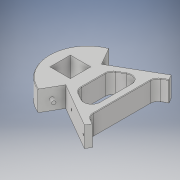
# Autodesk Inventor part: Profil_Winkel
Saved by Autodesk Inventor 2019 (Build 230136000, 136)
## iProperties
Created: 2018-08-17
Part Number: Profil_Winkel
Material: Generic
Document SubType Name: Modeling
Designer: Julia
Density: 1 g/cm^3
Appearance: Default
Author: Julia
Autodesk Inventor part; units mm, degrees
ref_plane "YZ Plane" through (0, 0, 0) normal (1, 0, 0) x (0, 1, 0)
ref_plane "XZ Plane" through (0, 0, 0) normal (0, 1, 0) x (-1, 0, 0)
ref_plane "XY Plane" through (0, 0, 0) normal (0, 0, 1) x (1, 0, 0)
sketch "Sketch1" plane through (0, 0, 0) normal (0, 1, 0) x (-1, 0, 0)
  line L0 (-126.3701, 48.161) -> (-51.2671, 4.8003) construction
  line L1 (-51.2671, 4.8003) -> (-126.3701, -38.5605) construction
  line L2 (-126.3701, -38.5605) -> (-126.3701, 48.161) construction
  line L3 (110.9585, 0) -> (-59.5814, 0) construction
  line L4 (83.2089, 69.641) -> (63.2089, 35)
  line L5 (63.2089, 35) -> (-23.3937, 85)
  line L6 (-23.3937, 85) -> (-29.3937, 74.6077)
  line L7 (-29.3937, 74.6077) -> (-12.0731, 64.6077)
  line L8 (0.9172, 57.1077) -> (44.2185, 32.1077)
  line L9 (83.2089, -69.641) -> (63.2089, -35)
  line L10 (63.2089, -35) -> (-23.3937, -85)
  line L11 (-23.3937, -85) -> (-29.3937, -74.6077)
  line L12 (-29.3937, -74.6077) -> (-12.0731, -64.6077)
  line L13 (0.9172, -57.1077) -> (44.2185, -32.1077)
  arc A0 (83.2089, -69.641) -> (83.2089, 69.641) centre (55.3678, 0) ccw
  line L14 (-12.0731, 64.6077) -> (-12.0731, -64.6077)
  line L15 (0.9172, 57.1077) -> (0.9172, -57.1077)
  line L16 (44.2185, 32.1077) -> (44.2185, -32.1077)
  dimension "d3" = 40
  dimension "d4" = 100
  dimension "d5" = 12
  dimension "d7" = 20
  dimension "d19" = 70
  dimension "d20" = 75
  dimension "d21" = 15
  dimension "d22" = 50
  constraints: 34 end point, 7 symmetric about line, 5 vertical, 4 perpendicular, 2 equal length, 2 horizontal, 2 point on circle, 1 centre point, 1 collinear, 1 parallel, 1 point on line, 3 other
  measures "d3" distance of L4.start L4.end
  measures "d4" distance of L4.end L5.end
  measures "d5" distance of L5.end L6.end
  measures "d7" distance of L6.end L7.end
  measures "d19" distance of L9.end L4.end
  measures "d20" radius of A0
  measures "d21" distance of L8.start L7.end
  measures "d22" distance of L8.start L8.end
extrude "Extrusion1" add sketch "Sketch1" along normal blind 40
sketch "Sketch2" plane through (-63.2089, 0, 35) normal (0.8660254, 0, 0.5) x (0.5, 0, -0.8660254)
  circle A0 centre (-20, 20) radius 3.4
  line L0 (-40, 40) -> (0, 40) projected
  line L1 (-40, 0) -> (-40, 40) projected
  point P0 (61.9153, 0)
  point P1 (-20, 40)
  point P2 (-40, 20)
  dimension "d10" = 6.8
  constraints: 2 midpoint, 1 centre point, 1 horizontal alignment, 1 vertical alignment
  measures "d10" diameter of A0
extrude "Extrusion2" add sketch "Sketch2" along normal blind 10
sketch "Sketch3" plane through (-83.2089, 0, -69.641) normal (0.8660254, 0, -0.5) x (-0.5, 0, -0.8660254)
  circle A0 centre (-20, 20) radius 3.4
  line L0 (-40, 40) -> (0, 40) projected
  line L1 (0, 0) -> (0, 40) projected
  point P0 (-101.9153, 0)
  point P1 (-20, 40)
  point P2 (0, 20)
  dimension "d13" = 6.8
  constraints: 2 midpoint, 1 centre point, 1 horizontal alignment, 1 vertical alignment
  measures "d13" diameter of A0
extrude "Extrusion3" add sketch "Sketch3" along normal blind 10
sketch "Sketch4" plane through (0, 40, 0) normal (0, 1, 0) x (1, 0, 0)
  line L0 (-109.2185, -20) -> (-69.2185, -20)
  line L1 (-69.2185, -20) -> (-69.2185, 20)
  line L2 (-69.2185, 20) -> (-109.2185, 20)
  line L3 (-109.2185, 20) -> (-109.2185, -20)
  line L4 (-44.2185, -32.1077) -> (-44.2185, 32.1077) projected
  point P0 (0, 0)
  point P1 (-109.2185, 0)
  dimension "d16" = 40
  dimension "d17" = 40
  dimension "d23" = 25
  constraints: 8 end point, 2 parallel, 1 horizontal, 1 horizontal alignment, 1 midpoint, 1 perpendicular
  measures "d16" distance of L2.end L0.start
  measures "d17" distance of L1.end L2.end
  measures "d23" distance between parallel lines of L1 L4
extrude "Extrusion4" cut sketch "Sketch4" against normal blind 40
fillet "Fillet1" radius 15 2 edges at (-44.2185, 20, -32.1077) (-44.2185, 20, 32.1077)
fillet "Fillet2" radius 15 2 edges at (-0.9172, 20, 57.1077) (-0.9172, 20, -57.1077)
fillet "Fillet3" radius 15 2 edges at (12.0731, 20, 64.6077) (12.0731, 20, -64.6077)
sketch "Sketch5" plane through (29.3937, 0, 74.6077) normal (0.5, 0, -0.8660254) x (-0.8660254, 0, -0.5)
  point P0 (62.7595, 0)
  point P1 (5.815, 19.918)
hole "Hole1" at (24.3577, 19.918, 71.7002) direction (-0.5, 0, 0.8660254) diameter 4 end through all counterbore diameter 5 counterbore depth 2
sketch "Sketch6" plane through (-36.7185, 0, 36.4378) normal (0.5, 0, -0.8660254) x (-0.8660254, 0, -0.5)
  point P0 (-13.5802, 0)
  point P1 (-7.7378, 18.9937)
hole "Hole2" at (-30.0174, 18.9937, 40.3067) direction (-0.5, 0, 0.8660254) diameter 4 end through all counterbore diameter 5 counterbore depth 2
fillet "Fillet8" radius 1 28 edges at (-42.2089, 0, 30.9474) (-30.0679, 0, 40.2776) (-8.4172, 0, 44.1173) (-0.9172, 0, 0) (-8.4172, 0, -44.1173) (-30.0679, 0, -40.2776) (-42.2089, 0, -30.9474) (-44.2185, 0, 0) (14.0828, 0, -63.4474) (24.4834, 0, -71.7728) (14.0828, 0, 63.4474) (24.4834, 0, 71.7728) (12.0731, 0, 0) (-42.2089, 40, -30.9474) (-30.0679, 40, -40.2776) (-8.4172, 40, -44.1173) (-0.9172, 40, 0) (-8.4172, 40, 44.1173) (-30.0679, 40, 40.2776) (-42.2089, 40, 30.9474) (-44.2185, 40, 0) (14.0828, 40, -63.4474) (24.4834, 40, -71.7728) (14.0828, 40, 63.4474) (24.4834, 40, 71.7728) (12.0731, 40, 0) (29.3937, 20, 74.6077) (29.3937, 20, -74.6077)
fillet "Fillet9" radius 1 2 edges at (-130.3678, 0, 0) (-130.3678, 40, 0)
body "Solid1"
